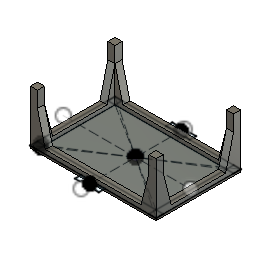
arduino_base (Autodesk Fusion 360 design; units mm, degrees)
Autodesk Fusion 360 part; units mm, degrees
sketch "Sketch1" plane through (0, 0, 0) normal (0, 1, 0) x (1, 0, 0)
  line L0 (-91.2966, 0) -> (69.6356, 0) construction
  line L1 (0, 61.5776) -> (0, -68.7711) construction
  line L2 (-79.5, -53.5) -> (-70.5, -53.5)
  line L3 (-70.5, -53.5) -> (-70.5, -44.5)
  line L4 (-70.5, -44.5) -> (-79.5, -44.5)
  line L5 (-79.5, -44.5) -> (-79.5, -53.5)
  line L6 (-79.5, 44.5) -> (-70.5, 44.5)
  line L7 (-70.5, 44.5) -> (-70.5, 53.5)
  line L8 (-70.5, 53.5) -> (-79.5, 53.5)
  line L9 (-79.5, 53.5) -> (-79.5, 44.5)
  line L10 (70.5, 44.5) -> (79.5, 44.5)
  line L11 (79.5, 44.5) -> (79.5, 53.5)
  line L12 (79.5, 53.5) -> (70.5, 53.5)
  line L13 (70.5, 53.5) -> (70.5, 44.5)
  line L14 (70.5, -53.5) -> (79.5, -53.5)
  line L15 (79.5, -53.5) -> (79.5, -44.5)
  line L16 (79.5, -44.5) -> (70.5, -44.5)
  line L17 (70.5, -44.5) -> (70.5, -53.5)
  line L18 (-79.5, 53.5) -> (79.5, 53.5)
  line L19 (79.5, 53.5) -> (79.5, -53.5)
  line L20 (79.5, -53.5) -> (-79.5, -53.5)
  line L21 (-79.5, -53.5) -> (-79.5, 53.5)
  line L22 (-79.5, 53.5) -> (79.5, -53.5) construction
  line L23 (79.5, 53.5) -> (-79.5, -53.5) construction
  line L24 (70.5, 44.5) -> (-70.5, 44.5)
  line L25 (-70.5, 44.5) -> (-70.5, -44.5)
  line L26 (-70.5, -44.5) -> (70.5, -44.5)
  line L27 (70.5, -44.5) -> (70.5, 44.5)
  line L28 (70.5, 44.5) -> (-70.5, -44.5) construction
  line L29 (-70.5, 44.5) -> (70.5, -44.5) construction
  line L30 (15, 53.5) -> (-15, 53.5)
  line L31 (-15, 53.5) -> (-15, 61.5)
  line L32 (-15, 61.5) -> (15, 61.5)
  line L33 (15, 61.5) -> (15, 53.5)
  line L34 (15, 53.5) -> (-15, 61.5) construction
  line L35 (-15, 53.5) -> (15, 61.5) construction
  line L36 (15, -53.5) -> (-15, -53.5)
  line L37 (-15, -53.5) -> (-15, -61.5)
  line L38 (-15, -61.5) -> (15, -61.5)
  line L39 (15, -61.5) -> (15, -53.5)
  line L40 (15, -53.5) -> (-15, -61.5) construction
  line L41 (-15, -53.5) -> (15, -61.5) construction
  point P0 (-75, -44.5)
  point P1 (-70.5, -49)
  point P2 (0, 57.5)
  point P3 (0, -57.5)
  dimension "d1" = 9
  dimension "d2" = 9
  dimension "d19" = 49
  dimension "d20" = 75
  dimension "d22" = 30
  dimension "d23" = 8
  constraint vertical L1
  constraint horizontal L0
  constraint coincident origin L0
  constraint coincident origin L1
  constraint horizontal L2
  constraint vertical L3
  constraint horizontal L4
  constraint vertical L5
  constraint horizontal L6
  constraint vertical L7
  constraint horizontal L8
  constraint vertical L9
  constraint horizontal L10
  constraint vertical L11
  constraint horizontal L12
  constraint vertical L13
  constraint horizontal L14
  constraint vertical L15
  constraint horizontal L16
  constraint vertical L17
  constraint symmetric L0 L2.start L8.end
  constraint symmetric L0 L3.end L6.end
  constraint symmetric L1 L8.end L11.end
  constraint symmetric L1 L6.end L10.start
  constraint symmetric L1 L2.start L14.end
  constraint symmetric L1 L3.end L16.end
  constraint horizontal L18
  constraint perpendicular L18 L19
  constraint parallel L18 L20
  constraint parallel L19 L21
  constraint coincident L22 origin
  constraint coincident L23 origin
  constraint coincident L1 origin
  constraint coincident L11.end L12.start
  constraint horizontal L24
  constraint perpendicular L24 L25
  constraint parallel L24 L26
  constraint parallel L25 L27
  constraint coincident L28 origin
  constraint coincident L29 origin
  constraint midpoint L4 P0
  constraint midpoint L3 P1
  constraint horizontal L30
  constraint perpendicular L30 L31
  constraint parallel L30 L32
  constraint parallel L31 L33
  constraint coincident L34 P2
  constraint coincident L35 P2
  constraint coincident L18 L30.start
  constraint coincident L1 P2
  constraint horizontal L36
  constraint perpendicular L36 L37
  constraint parallel L36 L38
  constraint parallel L37 L39
  constraint coincident L40 P3
  constraint coincident L41 P3
  constraint coincident L20 L36.start
  constraint coincident L1 P3
  constraint symmetric L0 L31.end L37.end
  measures "d1" distance of L2.start L2.end
  measures "d2" distance of L2.start L4.end
  measures "d19" distance of L0 P1
  measures "d20" distance of L1 P0
  measures "d22" distance of L31.end L32.end
  measures "d23" distance of L30.start L32.end
extrude "Extrude1" add sketch "Sketch1" against normal blind 3 contours L2 L3 L4 L5 L20 L21 | L3 L17 L20 L26 L36 | L4 L6 L21 L25 | L24 L25 L26 L27 | L6 L7 L8 L9 L18 L21 | L7 L13 L18 L24 L30 | L10 L16 L19 L27 | L14 L15 L16 L17 L19 L20 | L10 L11 L12 L13 L18 L19
extrude "Extrude2" add sketch "Sketch1" along normal blind 65 contours L2 L3 L4 L5 L20 L21 | L6 L7 L8 L9 L18 L21 | L14 L15 L16 L17 L19 L20 | L10 L11 L12 L13 L18 L19
extrude "Extrude3" add sketch "Sketch1" along normal blind 5 contours L3 L17 L20 L26 L36 | L4 L6 L21 L25 | L7 L13 L18 L24 L30 | L10 L16 L19 L27
chamfer "Chamfer1" distance 40 distance2 10 8 edges at (-75, 5, -44.5) (-75, 5, 44.5) (-70.5, 5, 49) (-70.5, 5, -49) (70.5, 5, -49) (75, 5, -44.5) (75, 5, 44.5) (70.5, 5, 49) measured on face at (-76.5, 45, -44.5) measured on face at (-73.5, 25, 44.5) measured on face at (-70.5, 25, 50.5) measured on face at (-70.5, 45, -47.5) measured on face at (70.5, 45, -47.5) measured on face at (73.5, 45, -44.5) measured on face at (76.5, 45, 44.5) measured on face at (70.5, 45, 50.5)
